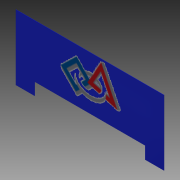
# Autodesk Inventor part: GE-13013BLogo
Saved by Autodesk Inventor 2013 (Build 170138000, 138)
## iProperties
Created: 2013-01-04
Part Number: GE-13013BLogo
Material: Polycarbonate, Clear
Document SubType Name: Modeling
Designer: Phillip
Density: 1 g/cm^3
Author: Phillip
Autodesk Inventor part; units mm, degrees
ref_plane "YZ Plane" through (0, 0, 0) normal (1, 0, 0) x (0, 1, 0)
ref_plane "XZ Plane" through (0, 0, 0) normal (0, 1, 0) x (-1, 0, 0)
ref_plane "XY Plane" through (0, 0, 0) normal (0, 0, 1) x (1, 0, 0)
sketch "Sketch1" plane through (0, 0, 0) normal (0, 0, 1) x (1, 0, 0)
  line L0 (0, 0) -> (1841.5, 0)
  line L1 (1841.5, 0) -> (1841.5, 812.8)
  line L2 (1841.5, 812.8) -> (1606.55, 812.8)
  line L3 (1606.55, 812.8) -> (1606.55, 660.4)
  line L4 (1606.55, 660.4) -> (234.95, 660.4)
  line L5 (234.95, 660.4) -> (234.95, 812.8)
  line L6 (234.95, 812.8) -> (0, 812.8)
  line L7 (0, 812.8) -> (0, 0)
  dimension "d0" = 1841.5
  dimension "d1" = 812.8
  dimension "d2" = 234.95
  dimension "d3" = 152.4
  dimension "d4" = 234.95
  dimension "d5" = 152.4
  constraints: 16 end point, 4 perpendicular, 3 parallel, 1 horizontal
  measures "d0" distance of L0.start L0.end
  measures "d1" distance of L0.end L1.end
  measures "d2" distance of L1.end L2.end
  measures "d3" distance of L2.end L3.end
  measures "d4" distance of L5.end L6.end
  measures "d5" distance between parallel lines of L6 L4
extrude "Extrusion1" add sketch "Sketch1" against normal blind 3.175
sketch "Sketch2" plane through (0, 0, 0) normal (0, 0, 1) x (1, 0, 0)
  line L0 (0, 0) -> (1841.5, 0) projected
  line L1 (1841.5, 0) -> (1841.5, 812.8) projected
  line L2 (1841.5, 812.8) -> (1606.55, 812.8) projected
  line L3 (1606.55, 812.8) -> (1606.55, 660.4) projected
  line L4 (1606.55, 660.4) -> (234.95, 660.4) projected
  line L5 (234.95, 660.4) -> (234.95, 812.8) projected
  line L6 (234.95, 812.8) -> (0, 812.8) projected
  line L7 (0, 812.8) -> (0, 0) projected
sketch "Sketch3" plane through (0, 0, 0) normal (0, 0, 1) x (1, 0, 0)
  line L0 (0, 0) -> (1841.5, 0) projected
  line L1 (521.4752, 0) -> (1320.0248, 0) construction
  line L2 (1320.0248, 0) -> (1320.0248, 559.6136) construction
  line L3 (1320.0248, 559.6136) -> (521.4752, 559.6136) construction
  line L4 (521.4752, 559.6136) -> (521.4752, 0) construction
  point P0 (920.75, 0)
  point P1 (920.75, 0)
  constraints: 2 midpoint, 1 coincident, 1 collinear, 1 horizontal, 2 other
decal "Decal1"
equation "\"d4\" = d2"
equation "\"d5\" = d3"
body "Solid1"
